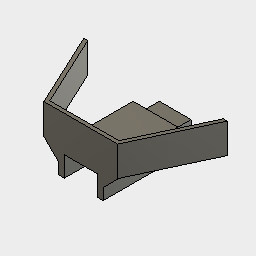
Front Cover v1 (Autodesk Fusion 360 design; units mm, degrees)
Autodesk Fusion 360 part; units mm, degrees
sketch "Sketch1" plane through (0, 0, 0) normal (0, 0, 1) x (1, 0, 0)
  line L0 (0, 0) -> (10.6, 0)
  line L1 (10.6, 0) -> (10.6, 6.6)
  line L2 (10.6, 6.6) -> (0, 6.6)
  line L3 (0, 6.6) -> (0, 0)
  dimension "d1" = 6.6
  dimension "d2" = 10.6
  constraint horizontal L0
  constraint vertical L1
  constraint horizontal L2
  constraint vertical L3
  constraint coincident L0.start L3.end
extrude "Extrude1" add sketch "Sketch1" along normal blind 6.6
sketch "Sketch2" plane through (0, 0, 6.6) normal (0, 0, 1) x (1, 0, 0)
  line L0 (0, 6.6) -> (0, 0)
  line L1 (0, 0) -> (10.6, 0)
  line L2 (10.6, 0) -> (10.6, 6.6)
  line L3 (10.6, 6.6) -> (0, 6.6)
  line L4 (0, 0) -> (-2.2, 0)
  line L5 (10.6, 0) -> (12.8, 0)
  line L6 (12.8, 0) -> (12.8, 8.8)
  line L7 (12.8, 8.8) -> (-2.2, 8.8)
  line L8 (-2.2, 8.8) -> (-2.2, 0)
  constraint coincident L0.end L1.start
  constraint parallel L2 L6
  constraint parallel L3 L7
  constraint parallel L0 L8
extrude "Extrude2" add sketch "Sketch2" along normal blind 25
sketch "Sketch6" plane through (0, 0, 31.6) normal (0, 0, 1) x (1, 0, 0)
  line L0 (-2.2, 0) -> (12.8, 0)
  line L1 (12.8, 0) -> (12.8, 8.8)
  line L2 (12.8, 8.8) -> (-2.2, 8.8)
  line L3 (-2.2, 8.8) -> (-2.2, 0)
  line L4 (-0.2, 2) -> (-0.2, 0)
  line L5 (10.8, 2) -> (10.8, 0)
  line L6 (10.8, 2) -> (10.8, 6.8)
  line L7 (10.8, 6.8) -> (-0.2, 6.8)
  line L8 (-0.2, 6.8) -> (-0.2, 2)
  dimension "d25" = 2
  dimension "d26" = 2
  constraint vertical L4
  constraint vertical L5
  constraint parallel L1 L6
  constraint parallel L2 L7
  constraint parallel L3 L8
extrude "Extrude7" cut sketch "Sketch6" against normal blind 7 contours L0 L4 L5 L6 L7 L8
sketch "Sketch7" plane through (0, 8.8, 0) normal (0, 1, 0) x (-1, 0, 0)
  line L0 (-12.8, 6.6) -> (2.2, 6.6)
  line L1 (2.2, 6.6) -> (2.2, 31.6)
  line L2 (2.2, 31.6) -> (-12.8, 31.6)
  line L3 (-12.8, 31.6) -> (-17.6423, 31.6)
  line L4 (-27.9759, 6.6) -> (-29.3, 6.6)
  line L5 (-17.6423, 31.6) -> (-29.3, 6.6)
  line L6 (-12.8, 30.4) -> (-16.8778, 30.4)
  line L7 (-16.8778, 30.4) -> (-27.4164, 7.8)
  line L8 (-27.4164, 7.8) -> (-27.9759, 6.6)
  line L9 (-12.8, 31.6) -> (-5.3, 31.6)
  line L10 (-12.8, 30.4) -> (-5.3, 30.4)
  line L11 (2.2, 30.4) -> (-5.3, 30.4)
  line L12 (2.2, 31.6) -> (-5.3, 31.6)
  line L13 (2.2, 31.6) -> (7.0423, 31.6)
  line L14 (2.2, 30.4) -> (6.2778, 30.4)
  line L15 (6.2778, 30.4) -> (16.8164, 7.8)
  line L16 (7.0423, 31.6) -> (18.7, 6.6)
  line L17 (17.3759, 6.6) -> (18.7, 6.6)
  line L18 (16.8164, 7.8) -> (17.3759, 6.6)
  constraint horizontal L3
  constraint parallel L3 L6
  constraint parallel L5 L7
  constraint parallel L7 L8
  constraint midpoint L2
  constraint parallel L15 L18
extrude "Extrude8" add sketch "Sketch7" along normal blind 10
chamfer "Chamfer2" distance 5 angle 45 2 edges at (12.8, 8.8, 31) (-2.2, 8.8, 31)
